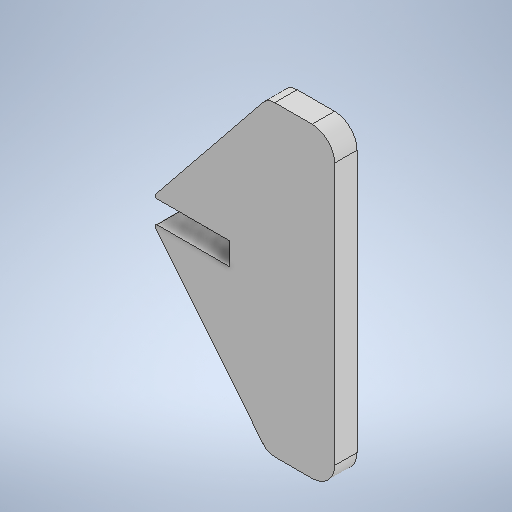
# Autodesk Inventor part: LEME
Saved by Autodesk Inventor 2025.1 (Build 291241000, 241)
## iProperties
Created: 2024-10-26
Part Number: LEME
Material: Genérico
Document SubType Name: Modeling
Designer: ambrosildo
Density: 1 g/cm^3
Appearance: Padrão
Author: ambrosildo
Autodesk Inventor part; units mm, degrees
ref_plane "YZ Plane" through (0, 0, 0) normal (1, 0, 0) x (0, 1, 0)
ref_plane "XZ Plane" through (0, 0, 0) normal (0, 1, 0) x (-1, 0, 0)
ref_plane "XY Plane" through (0, 0, 0) normal (0, 0, 1) x (1, 0, 0)
sketch "Esboço1" plane through (0, 0, 0) normal (0, 0, 1) x (1, 0, 0)
  line L0 (0, 0) -> (0, 17.5)
  arc A0 (0, 17.5) -> (-3, 20.5) centre (-3, 17.5) ccw
  line L1 (-3, 20.5) -> (-8, 20.5)
  arc A1 (-8, 20.5) -> (-9.5571, 19.7552) centre (-8, 18.5) ccw
  line L2 (-23.75, 1.5) -> (-14, 1.5)
  line L3 (-14, 1.5) -> (-14, 0)
  arc A2 (-23.9446, 1.9069) -> (-23.75, 1.5) centre (-23.75, 1.75) ccw
  line L4 (-23.9446, 1.9069) -> (-9.5571, 19.7552)
  line L5 (0, 0) -> (0, -17.5)
  arc A3 (-3, -20.5) -> (0, -17.5) centre (-3, -17.5) ccw
  line L6 (-3, -20.5) -> (-8, -20.5)
  arc A4 (-9.5571, -19.7552) -> (-8, -20.5) centre (-8, -18.5) ccw
  line L7 (-23.75, -1.5) -> (-14, -1.5)
  line L8 (-14, -1.5) -> (-14, 0)
  arc A5 (-23.75, -1.5) -> (-23.9446, -1.9069) centre (-23.75, -1.75) ccw
  line L9 (-23.9446, -1.9069) -> (-9.5571, -19.7552)
  point P0 (-7, 0)
  point P1 (-5.5, 20.5)
  point P2 (-5.5, -20.5)
  constraints: 20 end point, 12 point on circle, 6 centre point, 2 tangent, 2 vertical, 1 midpoint, 1 other
extrude "Extrusão1" add sketch "Esboço1" along normal blind 3
